DHECouletadapter (Autodesk Fusion 360 design; units mm, degrees)
Autodesk Fusion 360 part; units mm, degrees
sketch "Sketch1" plane through (0, 0, 0) normal (0, 1, 0) x (1, 0, 0)
  line L0 (47, 0) -> (47, -22)
  line L1 (47, -22) -> (45, -22)
  line L2 (45, -22) -> (45, -12)
  line L3 (45, -12) -> (35, -12)
  line L4 (35, -12) -> (35, -10)
  line L5 (35, -10) -> (45, -10)
  line L6 (45, -10) -> (45, 0)
  line L7 (45, 0) -> (47, 0)
  dimension "d1" = 45
  dimension "d2" = 35
  dimension "d3" = 2
  dimension "d4" = 2
  dimension "d5" = 10
  constraint vertical L0
  constraint perpendicular L0 L1
  constraint perpendicular L1 L2
  constraint perpendicular L2 L3
  constraint perpendicular L3 L4
  constraint perpendicular L4 L5
  constraint perpendicular L5 L6
  constraint perpendicular L0 L7
  constraint coincident origin L7
  constraint equal L2 L6
  constraint equal L1 L7
  measures "d1" distance of origin L6
  measures "d2" distance of origin L4
  measures "d3" distance of L0 L6
  measures "d4" distance of L3 L5
  measures "d5" distance of L5 L7
revolve "Revolve1" add sketch "Sketch1" angle 360 about axis through (0, 0, 1.75) along (0, 0, 1)
